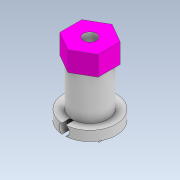
# Autodesk Inventor part: Coupling_0505_4.2
Saved by Autodesk Inventor 2022 (Build 260153000, 153)
## iProperties
Created: 2023-03-17
Part Number: Coupling_0505_4.2
Material: 一般
Document SubType Name: Modeling
Designer: JOU
Density: 1 g/cm^3
Appearance: 預設
Mass: 1.64153 g
Surface Area: 11.3377 cm^2
Volume: 1.64153 cm^3
Author: JOU
Title: 聯軸器
Autodesk Inventor part; units mm, degrees
ref_plane "YZ Plane" through (0, 0, 0) normal (1, 0, 0) x (0, 1, 0)
ref_plane "XZ Plane" through (0, 0, 0) normal (0, 1, 0) x (-1, 0, 0)
sketch "草圖1" plane through (0, 0, 0) normal (0, 1, 0) x (-1, 0, 0)
  circle A0 centre (0, 0) radius 5.5
  dimension "d0" = 11
  constraints: 1 centre point, 1 coincident
  measures "d0" diameter of A0
extrude "擠出1" add sketch "草圖1" along normal blind 16
sketch "草圖2" plane through (0, 16, 0) normal (0, 1, 0) x (1, 0, 0)
  line L0 (5.85, -3.3775) -> (0, -6.755)
  line L1 (0, -6.755) -> (-5.85, -3.3775)
  line L2 (-5.85, -3.3775) -> (-5.85, 3.3775)
  line L3 (-5.85, 3.3775) -> (0, 6.755)
  line L4 (0, 6.755) -> (5.85, 3.3775)
  line L5 (5.85, 3.3775) -> (5.85, -3.3775)
  point P0 (0, 0)
  point P1 (0, 0)
  dimension "d3" = 11.7
  constraints: 12 end point, 1 coincident, 1 vertical, 13 other
  measures "d3" distance between parallel lines of L5 L2
extrude "擠出2" add sketch "草圖2" along normal blind 6
sketch "草圖3" plane through (0, 0, 0) normal (0, -1, 0) x (1, 0, 0)
  circle A0 centre (0, 0) radius 1.95
  dimension "d6" = 3.9
  constraints: 1 centre point, 1 coincident
  measures "d6" diameter of A0
extrude "擠出3" cut sketch "草圖3" against normal up to surface (22 mm away)
sketch "草圖19" plane through (0, 0, 0) normal (0, -1, 0) x (1, 0, 0)
  circle A0 centre (0, 0) radius 8
  circle A1 centre (0, 0) radius 5.5 projected
  dimension "d56" = 16
  constraints: 1 centre point, 1 coincident
  measures "d56" diameter of A0
extrude "擠出17" add sketch "草圖19" against normal blind 3
sketch "草圖20" plane through (0, 0, 0) normal (0, -1, 0) x (1, 0, 0)
  line L0 (1.25, -1.4967) -> (-1.25, -1.4967)
  line L1 (-1.25, -1.4967) -> (-1.25, -3.2967)
  line L2 (-1.25, -3.2967) -> (1.25, -3.2967)
  line L3 (1.25, -3.2967) -> (1.25, -1.4967)
  circle A0 centre (0, 0) radius 1.95 projected
  dimension "d59" = 1.8
  dimension "d60" = 2.5
  constraints: 8 end point, 2 parallel, 2 point on circle, 1 horizontal, 1 perpendicular
  measures "d59" distance of L0.end L1.end
  measures "d60" distance of L1.end L2.end
extrude "擠出18" add sketch "草圖20" along normal blind 6 contours L3 L2 L1 A0
ref_plane "工作平面4" through (0, 0, 8) normal (0, 0, 1) x (1, 0, 0)
sketch "草圖21" plane through (0, 0, 8) normal (0, 0, 1) x (1, 0, 0)
  circle A0 centre (0, 1.5) radius 1.5
  line L0 (0, -4.4) -> (0, 26.4) projected
  line L1 (-8, 0) -> (8, 0) projected
  point P0 (0, 0)
  dimension "d63" = 3
  dimension "d64" = 1.5
  constraints: 1 centre point, 1 point on line
  measures "d63" diameter of A0
  measures "d64" distance from line of L1 A0.centre
extrude "擠出19" cut sketch "草圖21" against normal up to surface round surface about axis through (0, 0, 0) along (0, 1, 0) radius 1.95 far side no
sketch "草圖22" plane through (0, 0, 8) normal (0, 0, 1) x (1, 0, 0)
  line L0 (0, -4.52) -> (0, 26.42) projected
  circle A0 centre (0, 1.5) radius 1.6
  line L1 (-8, 0) -> (8, 0) projected
  point P0 (0, 0)
  dimension "d67" = 1.5
  dimension "d68" = 3.2
  constraints: 1 centre point, 1 point on line
  measures "d67" distance from line of L1 A0.centre
  measures "d68" diameter of A0
extrude "擠出20" cut sketch "草圖22" against normal up to surface round surface about axis through (0, 0, 0) along (0, 1, 0) radius 5.5 far side no
